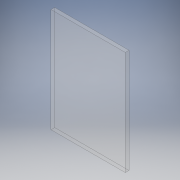
# Autodesk Inventor part: toppoly
Saved by Autodesk Inventor 2017 (Build 210142000, 142)
## iProperties
Created: 2017-08-02
Part Number: toppoly
Material: Polycarbonate, Clear
Document SubType Name: Modeling
Designer: Kai
Density: 1.2 g/cm^3
Appearance: Polycarbonate - Clear
Author: Kai
Autodesk Inventor part; units mm, degrees
ref_plane "YZ Plane" through (0, 0, 0) normal (1, 0, 0) x (0, 1, 0)
ref_plane "XZ Plane" through (0, 0, 0) normal (0, 1, 0) x (-1, 0, 0)
ref_plane "XY Plane" through (0, 0, 0) normal (0, 0, 1) x (1, 0, 0)
sketch "Sketch1" plane through (0, 0, 0) normal (0, 0, 1) x (1, 0, 0)
  line L0 (0, 0) -> (-254, 0)
  line L1 (-254, 0) -> (-254, 355.6)
  line L2 (-254, 355.6) -> (0, 355.6)
  line L3 (0, 355.6) -> (0, 0)
  dimension "d0" = 254
  dimension "d1" = 355.6
  constraints: 8 end point, 2 parallel, 1 horizontal, 1 perpendicular
  measures "d0" distance of L1.end L2.end
  measures "d1" distance of L0.end L1.end
extrude "Extrusion1" add sketch "Sketch1" along normal blind 12.7
body "Solid1"
